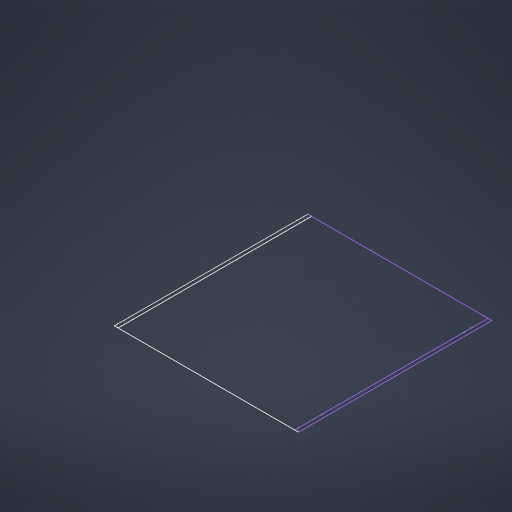
# Autodesk Inventor part: Деталь1
Saved by Autodesk Inventor 2023.4 (Build 274418000, 418)
## iProperties
Created: 2026-09-26
Part Number: Деталь1
Material: Типовые
Document SubType Name: Modeling
Designer: desig
Density: 1 g/cm^3
Appearance: По умолчанию
Author: desig
Autodesk Inventor part; units mm, degrees
ref_plane "YZ Plane" through (0, 0, 0) normal (1, 0, 0) x (0, 1, 0)
ref_plane "XZ Plane" through (0, 0, 0) normal (0, 1, 0) x (-1, 0, 0)
ref_plane "XY Plane" through (0, 0, 0) normal (0, 0, 1) x (1, 0, 0)
sketch "Эскиз1" plane through (0, 0, 0) normal (0, 1, 0) x (-1, 0, 0)
  line L0 (0, 0) -> (-16, 0)
  line L1 (-16, 0) -> (-16, -824.5203)
  line L2 (-16, -824.5203) -> (0, -824.5203)
  line L3 (0, -824.5203) -> (0, 0)
  line L4 (-769.0334, 0) -> (-785.0334, 0)
  line L5 (-785.0334, 0) -> (-785.0334, -824.5203)
  line L6 (-785.0334, -824.5203) -> (-769.0334, -824.5203)
  line L7 (-769.0334, -824.5203) -> (-769.0334, 0)
  line L8 (-16, -824.5203) -> (-769.0334, -824.5203)
  line L9 (-16, 0) -> (-769.0334, 0)
  dimension "d0" = 16
  dimension "d1" = 16
  dimension "d46" = 824.52
  dimension "d47" = 785.033
  constraints: 20 end point, 4 parallel, 3 horizontal, 3 perpendicular, 2 point on line
  measures "d0" distance of L1.end L2.end
  measures "d1" distance of L5.end L6.end
  measures "d46" distance of L2.end L0.start
  measures "d47" distance between parallel lines of L5 L3
extrude "Выдавливание1" add sketch "Эскиз1" along normal blind 500 contours L3 L2 L1 L0
extrude "Выдавливание2" add sketch "Эскиз1" against normal blind 16 from surface at 500 separate body contours L1 L8 L7 L9
extrude "Выдавливание3" add sketch "Эскиз1" along normal blind 16 separate body contours L1 L8 L7 L9
extrude "Выдавливание4" add sketch "Эскиз1" along normal up to surface (500 mm away) separate body contours L7 L6 L5 L4
sketch "DrillingSketch_1" plane through (16, 484, 0) normal (-1, 0, 0) x (0, 0, 1)
  line L0 (0, 0) -> (-824.5203, 0) projected
  line L1 (0, 16) -> (0, 0) projected
  line L2 (0, 16) -> (-824.5203, 16) projected
  line L3 (-824.5203, 0) -> (-824.5203, 16) projected
  line L4 (0, 8) -> (-824.5203, 8) construction
  line L5 (-412.2601, 8) -> (-412.2601, -12) construction
  point P0 (-76.2601, 8)
  point P1 (-748.2601, 8)
  point P2 (-108.2601, 8)
  point P3 (-716.2601, 8)
  dimension "d5" = 16
  dimension "Минимальный_отступ_присадки_от_кромки_Каркас" = 70
  dimension "Long_edge_1" = 824.5203
  dimension "Расстояние_между_точками" = 672
  dimension "d1107" = 32
  constraints: 5 point on line, 4 end point, 4 midpoint, 2 symmetric about line, 1 perpendicular
  measures "Long_edge_1" distance of L4.start L4.end
  measures "Расстояние_между_точками" distance of point (-748.26, 8) point (-76.26, 8)
  measures "d1107" distance of point (-76.26, 8) point (-108.26, 8)
sketch "DrillingSketch_2" plane through (769.0334, 0, 0) normal (1, 0, 0) x (0, 0, -1)
  line L0 (0, 0) -> (824.5203, 0) projected
  line L1 (824.5203, 0) -> (824.5203, 16) projected
  line L2 (0, 16) -> (824.5203, 16) projected
  line L3 (0, 0) -> (0, 16) projected
  line L4 (824.5203, 8) -> (0, 8) construction
  line L5 (412.2601, 8) -> (412.2601, -12) construction
  point P0 (748.2601, 8)
  point P1 (76.2601, 8)
  point P2 (716.2601, 8)
  point P3 (108.2601, 8)
  dimension "Минимальный_отступ_присадки_от_кромки_Каркас" = 70
  dimension "Long_edge_2" = 824.5203
  dimension "Расстояние_между_точками_2" = 672
  dimension "d1110" = 32
  constraints: 5 point on line, 4 end point, 4 midpoint, 2 symmetric about line, 1 perpendicular
  measures "Long_edge_2" distance of L4.start L4.end
  measures "Расстояние_между_точками_2" distance of point (76.26, 8) point (748.26, 8)
  measures "d1110" distance of point (748.26, 8) point (716.26, 8)
sketch "DrawerSketch_1" plane through (769.0334, 484, -824.5203) normal (1, 0, 0) x (0, 0, -1)
  line L0 (0, 0) -> (-824.5203, 0) projected
  line L1 (0, 0) -> (0, 16) projected
  line L2 (0, 16) -> (-824.5203, 16) projected
  line L3 (-824.5203, 0) -> (-824.5203, 16) projected
  line L4 (0, 8) -> (-824.5203, 8) construction
  line L5 (-412.2601, 8) -> (-412.2601, -12) construction
  point P0 (-28.2601, 8)
  point P1 (-796.2601, 8)
  point P2 (-60.2601, 8)
  point P3 (-764.2601, 8)
  dimension "d46" = 824.52
  dimension "d47" = 785.033
  dimension "Минимальный_отступ_присадки_от_кромки_Ящик" = 20
  dimension "Long_edge_1_2" = 824.5203
  dimension "Расстояние_между_точками_3" = 768
  dimension "d1113" = 32
  constraints: 5 point on line, 4 end point, 4 midpoint, 2 symmetric about line, 1 perpendicular
  measures "Long_edge_1_2" distance of L4.start L4.end
  measures "Расстояние_между_точками_3" distance of point (-796.26, 8) point (-28.26, 8)
  measures "d1113" distance of point (-28.26, 8) point (-60.26, 8)
sketch "DrawerSketch_2" plane through (16, 0, -824.5203) normal (-1, 0, 0) x (0, 0, 1)
  line L0 (0, 0) -> (824.5203, 0) projected
  line L1 (824.5203, 0) -> (824.5203, 16) projected
  line L2 (0, 16) -> (824.5203, 16) projected
  line L3 (0, 0) -> (0, 16) projected
  line L4 (824.5203, 8) -> (0, 8) construction
  line L5 (412.2601, 8) -> (412.2601, -12) construction
  point P0 (796.2601, 8)
  point P1 (28.2601, 8)
  point P2 (764.2601, 8)
  point P3 (60.2601, 8)
  dimension "d46" = 824.52
  dimension "d47" = 785.033
  dimension "Минимальный_отступ_присадки_от_кромки_Ящик" = 20
  dimension "Long_edge_2_2" = 824.5203
  dimension "Расстояние_между_точками_4" = 768
  dimension "d1116" = 32
  constraints: 5 point on line, 4 end point, 4 midpoint, 2 symmetric about line, 1 perpendicular
  measures "Long_edge_2_2" distance of L4.start L4.end
  measures "Расстояние_между_точками_4" distance of point (28.26, 8) point (796.26, 8)
  measures "d1116" distance of point (796.26, 8) point (764.26, 8)
hole "Stiajka outer 8x34" at (769.0334, 8, -748.2601) at (769.0334, 8, -76.2601) direction (-1, 0, 0) diameter 8 depth 34 bodies 1 2 3 4
hole "Stiajka outer 5x13" at (769.0334, 8, -748.2601) at (769.0334, 8, -76.2601) direction (1, 0, 0) diameter 5 depth 12.5 bodies 1 2 3 4
hole "Shkant 8x10" at (769.0334, 8, -716.2601) at (769.0334, 8, -108.2601) direction (1, 0, 0) diameter 8 depth 10 bodies 1 2 3 4
hole "Shkant 8x20" at (769.0334, 8, -716.2601) at (769.0334, 8, -108.2601) direction (-1, 0, 0) diameter 8 depth 20 bodies 1 2 3 4
sketch "StiajkaSideSketch" plane through (0, 0, 0) normal (0, -1, 0) x (1, 0, 0)
  line L0 (769.0334, -744.2601) -> (769.0334, -752.2601) projected
  line L1 (735.0334, -752.2601) -> (735.0334, -744.2601) projected
  line L2 (769.0334, -72.2601) -> (769.0334, -80.2601) projected
  line L3 (735.0334, -80.2601) -> (735.0334, -72.2601) projected
  point P0 (735.0334, -748.2601)
  point P1 (735.0334, -76.2601)
  dimension "d46" = 824.52
  dimension "d47" = 785.033
  constraints: 2 midpoint
hole "Stiajka cup" at (735.0334, 0, -748.2601) at (735.0334, 0, -76.2601) direction (0, 1, 0) diameter 15 depth 12.5 bodies 1 2 3 4
hole "Stiajka outer 8x34 2" at (769.0334, 492, -796.2601) at (769.0334, 492, -28.2601) direction (-1, 0, 0) diameter 8 depth 34 bodies 1 2 3 4
hole "Stiajka outer 5x13 2" at (769.0334, 492, -796.2601) at (769.0334, 492, -28.2601) direction (1, 0, 0) diameter 5 depth 12.5 bodies 1 2 3 4
hole "Shkant 8x10 2" at (769.0334, 492, -764.2601) at (769.0334, 492, -60.2601) direction (1, 0, 0) diameter 8 depth 10 bodies 1 2 3 4
hole "Shkant 8x20 2" at (769.0334, 492, -764.2601) at (769.0334, 492, -60.2601) direction (-1, 0, 0) diameter 8 depth 20 bodies 1 2 3 4
sketch "StiajkaSideSketch_2" plane through (16, 484, 0) normal (0, -1, 0) x (1, 0, 0)
  line L0 (753.0334, -792.2601) -> (753.0334, -800.2601) projected
  line L1 (719.0334, -800.2601) -> (719.0334, -792.2601) projected
  line L2 (753.0334, -24.2601) -> (753.0334, -32.2601) projected
  line L3 (719.0334, -32.2601) -> (719.0334, -24.2601) projected
  point P0 (719.0334, -796.2601)
  point P1 (719.0334, -28.2601)
  dimension "d46" = 824.52
  dimension "d47" = 785.033
  constraints: 2 midpoint
hole "Stiajka cup 2" at (735.0334, 484, -796.2601) at (735.0334, 484, -28.2601) direction (0, 1, 0) diameter 15 depth 12.5 bodies 1 2 3 4
hole "Stiajka outer 8x34 3" at (16, 8, -28.2601) at (16, 8, -796.2601) direction (1, 0, 0) diameter 8 depth 34 bodies 1 2 3 4
hole "Stiajka outer 5x13 3" at (16, 8, -28.2601) at (16, 8, -796.2601) direction (-1, 0, 0) diameter 5 depth 12.5 bodies 1 2 3 4
hole "Shkant 8x10 3" at (16, 8, -60.2601) at (16, 8, -764.2601) direction (-1, 0, 0) diameter 8 depth 10 bodies 1 2 3 4
hole "Shkant 8x20 3" at (16, 8, -60.2601) at (16, 8, -764.2601) direction (1, 0, 0) diameter 8 depth 20 bodies 1 2 3 4
sketch "StiajkaSideSketch_3" plane through (0, 0, 0) normal (0, -1, 0) x (1, 0, 0)
  line L0 (16, -32.2601) -> (16, -24.2601) projected
  line L1 (50, -24.2601) -> (50, -32.2601) projected
  line L2 (16, -800.2601) -> (16, -792.2601) projected
  line L3 (50, -792.2601) -> (50, -800.2601) projected
  point P0 (50, -28.2601)
  point P1 (50, -796.2601)
  dimension "d46" = 824.52
  dimension "d47" = 785.033
  constraints: 2 midpoint
hole "Stiajka cup 3" at (50, 0, -28.2601) at (50, 0, -796.2601) direction (0, 1, 0) diameter 15 depth 12.5 bodies 1 2 3 4
hole "Confirmat 5mm inward" at (16, 492, -76.2601) at (16, 492, -412.2601) at (16, 492, -748.2601) direction (-1, 0, 0) diameter 5 depth 20 bodies 1 2 3 4
hole "Confirmat 3mm outward" at (16, 492, -76.2601) at (16, 492, -412.2601) at (16, 492, -748.2601) direction (1, 0, 0) diameter 3 depth 35 bodies 1 2 3 4
equation "\"d0\" = Толщина_каркаса"
equation "\"d1\" = Толщина_каркаса"
equation "\"d5\" = Толщина_каркаса"
equation "\"d7\" = Толщина_каркаса"
equation "\"Минимальный_отступ_присадки_от_кромки_Каркас\" = 70"
equation "\"Минимальный_отступ_присадки_от_кромки_Ящик\" = 20"
equation "\"Толщина_каркаса\" = 16"
equation "\"Стяжка_D\" = 15"
equation "\"Стяжка_h\" = 12.5"
equation "\"Стяжка_D_резьбыШтока\" = 5"
equation "\"Стяжка_D_телаШтока\" = 8"
equation "\"Стяжка_резьбыШтока_Петля_h\" = 12.5"
equation "\"Стяжка_отступ\" = 34"
equation "\"Конфирмат_D_вПласть\" = 8"
equation "\"Конфирмат_D_вТорец\" = 5"
equation "\"Толщина_каркаса_ящика\" = 16"
equation "\"Шкант_D\" = 8"
equation "\"Полкодержатель_D\" = 5"
equation "\"Полкодержатель_смещение_от_низа_полки\" = 5"
equation "\"Петля_D_присадки\" = 35"
equation "\"M_Конфирмат_глубина_резьбы\" = 35"
equation "\"M_Конфирмат_D_вПласть\" = 5"
equation "\"M_Конфирмат_D_вТорец\" = 3"
equation "\"Толщина_задн_ст_Володя\" = 3"
equation "\"Толщина_дна_ящика_Володя\" = 6"
equation "\"Минимальное_расстояния_от_заднСт_ящика_до_заднСт\" = 25"
equation "\"Западание_кромки_полки_за_каркас\" = 5"
